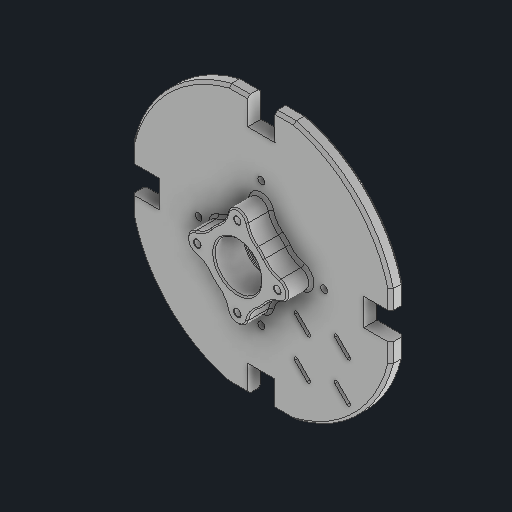
# Autodesk Inventor part: plate_lower
Saved by Autodesk Inventor 2027.1 (Build 311270010, 270A)
## iProperties
Created: 2026-10-07
Part Number: plate_lower
Material: Generisch
Document SubType Name: Modeling
Designer: luca
Density: 1 g/cm^3
Appearance: Vorgabe
Author: luca
## iProperties of the stored document plate_middle_3DPrint.ipt
Created: 2026-10-13
Part Number: plate_middle_3DPrint
Material: Generic
Document SubType Name: Modeling
Designer: lucao
Density: 1 g/cm^3
Appearance: Default
Author: lucao
Autodesk Inventor part; units mm, degrees
ref_plane "YZ Plane" through (0, 0, 0) normal (1, 0, 0) x (0, 1, 0)
ref_plane "XZ Plane" through (0, 0, 0) normal (0, 1, 0) x (-1, 0, 0)
ref_plane "XY Plane" through (0, 0, 0) normal (0, 0, 1) x (1, 0, 0)
sketch "Skizze1" plane through (0, 0, 0) normal (0, 1, 0) x (-1, 0, 0)
  circle A0 centre (0, 0) radius 100
  dimension "d0" = 200
  constraints: 1 centre point, 1 coincident
  measures "d0" diameter of A0
extrude "Extrusion1" add sketch "Skizze1" along normal blind 10
sketch "Skizze2" plane through (0, 10, 0) normal (0, 1, 0) x (1, 0, 0)
  circle A0 centre (0, 0) radius 100 projected
  circle A1 centre (-87, 0) radius 3.1
  dimension "d3" = 6.2
  dimension "d4" = 87
  dimension "d5" = 200
  constraints: 1 centre point, 1 horizontal alignment
  measures "d3" diameter of A1
  measures "d4" distance of A1.centre A0.centre
  measures "d5" diameter of A0
extrude "Extrusion2" cut sketch "Skizze2" against normal through all contours A1
chamfer "Fasen1" distance 3 angle 45 1 edges at (-90.1, 0, 0)
sketch "Skizze3" plane through (0, 10, 0) normal (0, 1, 0) x (1, 0, 0)
  circle A0 centre (-87, 0) radius 3.1 projected
  circle A1 centre (0, 0) radius 100 projected
  line L0 (-97, -24.3105) -> (-97, 24.3105)
  circle A2 centre (0, 0) radius 100 projected
  point P0 (-97, -24.3105)
  dimension "d11" = 10
  constraints: 2 end point, 1 point on circle, 1 vertical, 2 other
  measures "d11" distance from line of A0.centre L0
extrude "Extrusion3" cut sketch "Skizze3" against normal through all contours L0 A1 picked at (-97.7491, 4.0825)
pattern_circular "Runde Anordnung3" count 4 over 360 about axis through (0, -10, 0) along (0, 1, 0) of "Extrusion2", "Fasen1"
pattern_circular "Runde Anordnung4" count 4 over 360 about axis through (0, -10, 0) along (0, 1, 0) of "Extrusion3"
sketch "Skizze4" plane through (0, 0, 0) normal (0, -1, 0) x (1, 0, 0)
  circle A0 centre (0, 0) radius 15
  dimension "d26" = 30
  constraints: 1 centre point, 1 coincident
  measures "d26" diameter of A0
extrude "Extrusion4" cut sketch "Skizze4" against normal through all
sketch "Skizze5" plane through (0, 0, 0) normal (0, -1, 0) x (1, 0, 0)
  circle A0 centre (0, 0) radius 15 projected
  circle A1 centre (0, -87) radius 6.1 projected
  circle A2 centre (0, 87) radius 6.1 projected
  line L0 (-24.3105, -97) -> (24.3105, -97) projected
  arc A3 (24.3105, -97) -> (97, -24.3105) centre (0, 0) ccw projected
  line L1 (97, -24.3105) -> (97, 24.3105) projected
  arc A4 (97, 24.3105) -> (24.3105, 97) centre (0, 0) ccw projected
  line L2 (24.3105, 97) -> (-24.3105, 97) projected
  arc A5 (-24.3105, 97) -> (-97, 24.3105) centre (0, 0) ccw projected
  line L3 (-97, 24.3105) -> (-97, -24.3105) projected
  arc A6 (-97, -24.3105) -> (-24.3105, -97) centre (0, 0) ccw projected
  circle A7 centre (-87, 0) radius 6.1 projected
  circle A8 centre (87, 0) radius 6.1 projected
  line L4 (-10.25, 76.75) -> (10.25, 76.75)
  line L5 (10.25, 76.75) -> (10.25, 97.25)
  line L6 (10.25, 97.25) -> (-10.25, 97.25)
  line L7 (-10.25, 97.25) -> (-10.25, 76.75)
  line L8 (-10.25, 76.75) -> (10.25, 97.25) construction
  line L9 (10.25, 76.75) -> (-10.25, 97.25) construction
  point P0 (10.25, 97)
  point P1 (-10.25, 97)
  dimension "d29" = 20.5
  dimension "d30" = 20.5
  constraints: 12 end point, 2 midpoint, 2 parallel, 1 horizontal, 1 perpendicular
  measures "d29" distance of L6.end L5.end
  measures "d30" distance of L5.end L4.end
extrude "Extrusion5" cut sketch "Skizze5" against normal through all contours A2 | L2 L5 L4 L7
pattern_circular "Runde Anordnung5" count 4 over 360 about axis through (0, 0, 0) along (0, 1, 0) of "Extrusion5"
sketch "Sketch10" plane through (0, 0, 0) normal (0, -1, 0) x (1, 0, 0)
  circle A0 centre (0, 0) radius 25
  circle A1 centre (0, 0) radius 15 projected
  dimension "d63" = 50
  constraints: 1 centre point, 1 coincident
  measures "d63" diameter of A0
extrude "Extrusion9" add sketch "Sketch10" along normal blind 18
sketch "Sketch11" plane through (0, -18, 0) normal (0, -1, 0) x (1, 0, 0)
  circle A0 centre (0, 0) radius 17.525
  dimension "d66" = 35.05
  constraints: 1 centre point, 1 coincident
  measures "d66" diameter of A0
extrude "Extrusion10" cut sketch "Sketch11" against normal through all
sketch "Sketch12" plane through (0, 0, 0) normal (0, -1, 0) x (1, 0, 0)
  circle A0 centre (0, 0) radius 17.525 projected
  circle A1 centre (0, 0) radius 25 projected
  circle A2 centre (0, -30) radius 2.55
  circle A3 centre (0, -30) radius 7.5
  arc A4 (14.8914, -20.081) -> (7.3103, -31.6761) centre (26.8045, -36.1458) ccw
  arc A5 (-7.3103, -31.6761) -> (-14.8914, -20.081) centre (-26.8045, -36.1458) ccw
  dimension "d69" = 5.1
  dimension "d70" = 30
  dimension "d71" = 15
  dimension "d72" = 20
  dimension "d73" = 20
  constraints: 8 point on circle, 4 centre point, 4 tangent, 1 coincident, 1 vertical alignment
  measures "d69" diameter of A2
  measures "d70" distance of point (0, 0) A2.centre
  measures "d71" diameter of A3
  measures "d72" radius of A4
  measures "d73" radius of A5
extrude "Extrusion11" add sketch "Sketch12" along normal up to surface (18 mm away) contours A1 A3 A5 | A4 A3 A1 | A1 A3 picked at (2.8959, -25.9101)
pattern_circular "Circular Pattern6" count 4 over 360 about axis through (0, -18, 0) along (0, 1, 0) of "Extrusion11"
sketch "Sketch13" plane through (0, 10, 0) normal (0, 1, 0) x (1, 0, 0)
  circle A0 centre (0, 0) radius 17.525 projected
  circle A1 centre (0, 0) radius 15
  dimension "d79" = 30
  constraints: 1 centre point, 1 coincident
  measures "d79" diameter of A1
extrude "Extrusion12" add sketch "Sketch13" against normal blind 3
sketch "Sketch14" plane through (0, -18, 0) normal (0, -1, 0) x (1, 0, 0)
  circle A0 centre (30, 0) radius 2.55 projected
  circle A1 centre (0, 30) radius 2.55 projected
  circle A2 centre (-30, 0) radius 2.55 projected
  circle A3 centre (0, -30) radius 2.55 projected
  circle A4 centre (0, 0) radius 17.525 projected
  arc A5 (14.8914, -20.081) -> (20.081, -14.8914) centre (0, 0) ccw projected
  arc A6 (31.6761, -7.3103) -> (20.081, -14.8914) centre (36.1458, -26.8045) ccw projected
  arc A7 (31.6761, -7.3103) -> (31.6761, 7.3103) centre (30, 0) ccw projected
  arc A8 (20.081, 14.8914) -> (31.6761, 7.3103) centre (36.1458, 26.8045) ccw projected
  arc A9 (20.081, 14.8914) -> (14.8914, 20.081) centre (0, 0) ccw projected
  arc A10 (7.3103, 31.6761) -> (14.8914, 20.081) centre (26.8045, 36.1458) ccw projected
  arc A11 (7.3103, 31.6761) -> (-7.3103, 31.6761) centre (0, 30) ccw projected
  arc A12 (-14.8914, 20.081) -> (-7.3103, 31.6761) centre (-26.8045, 36.1458) ccw projected
  arc A13 (-14.8914, 20.081) -> (-20.081, 14.8914) centre (0, 0) ccw projected
  arc A14 (-31.6761, 7.3103) -> (-20.081, 14.8914) centre (-36.1458, 26.8045) ccw projected
  arc A15 (-31.6761, 7.3103) -> (-31.6761, -7.3103) centre (-30, 0) ccw projected
  arc A16 (-20.081, -14.8914) -> (-31.6761, -7.3103) centre (-36.1458, -26.8045) ccw projected
  arc A17 (-20.081, -14.8914) -> (-14.8914, -20.081) centre (0, 0) ccw projected
  arc A18 (-7.3103, -31.6761) -> (-14.8914, -20.081) centre (-26.8045, -36.1458) ccw projected
  arc A19 (-7.3103, -31.6761) -> (7.3103, -31.6761) centre (0, -30) ccw projected
  arc A20 (14.8914, -20.081) -> (7.3103, -31.6761) centre (26.8045, -36.1458) ccw projected
extrude "Extrusion13" cut sketch "Sketch14" against normal through all contours A0 | A1 | A2 | A3
sketch "Sketch15" plane through (0, 0, 0) normal (0, -1, 0) x (1, 0, 0)
  line L0 (0, 0) -> (70.7107, -70.7107) construction
  arc A0 (24.3105, -97) -> (97, -24.3105) centre (0, 0) ccw projected
  line L1 (0, 0) -> (0, -76.75) construction
  circle A1 centre (56.163, -56.163) radius 1.55
  circle A2 centre (26.163, -26.163) radius 1.55
  circle A3 centre (56.163, -26.163) radius 1.55
  circle A4 centre (26.163, -56.163) radius 1.55
  line L2 (26.163, -26.163) -> (56.163, -26.163) construction
  line L3 (56.163, -26.163) -> (56.163, -56.163) construction
  line L4 (56.163, -56.163) -> (26.163, -56.163) construction
  line L5 (26.163, -56.163) -> (26.163, -26.163) construction
  line L6 (26.163, -56.163) -> (35.3553, -65.3553) construction
  line L7 (56.163, -26.163) -> (65.3553, -35.3553) construction
  circle A5 centre (65.3553, -65.3553) radius 1.55
  circle A6 centre (65.3553, -35.3553) radius 1.55
  circle A7 centre (35.3553, -65.3553) radius 1.55
  circle A8 centre (35.3553, -35.3553) radius 1.55
  line L8 (55.0669, -57.259) -> (64.2593, -66.4514)
  line L9 (66.4514, -64.2593) -> (57.259, -55.0669)
  line L10 (34.2593, -66.4514) -> (25.0669, -57.259)
  line L11 (27.259, -55.0669) -> (36.4514, -64.2593)
  line L12 (34.2593, -36.4514) -> (25.0669, -27.259)
  line L13 (27.259, -25.0669) -> (36.4514, -34.2593)
  line L14 (55.0669, -27.259) -> (64.2593, -36.4514)
  line L15 (66.4514, -34.2593) -> (57.259, -25.0669)
  line L16 (-10.25, -76.75) -> (10.25, -76.75) projected
  dimension "d84" = 45
  dimension "d85" = 3.1
  dimension "d86" = 3.1
  dimension "d87" = 3.1
  dimension "d88" = 3.1
  dimension "d89" = 30
  dimension "d90" = 37
  dimension "d93" = 13
  dimension "d94" = 13
  dimension "d95" = 3.1
  dimension "d96" = 3.1
  dimension "d97" = 13
  dimension "d98" = 3.1
  dimension "d99" = 3.1
  dimension "d100" = 13
  constraints: 32 end point, 17 point on circle, 13 tangent, 8 centre point, 6 parallel, 3 coincident, 3 point on line, 2 midpoint, 1 horizontal, 1 perpendicular, 1 vertical
  measures "d84" angle of L0 L1
  measures "d85" diameter of A1
  measures "d86" diameter of A2
  measures "d87" diameter of A3
  measures "d88" diameter of A4
  measures "d89" distance of L3.end L4.end
  measures "d90" distance of L0.start L2.start
  measures "d93" distance of L4.end L6.end
  measures "d94" distance of L2.end L7.end
  measures "d95" diameter of A5
  measures "d96" diameter of A6
  measures "d97" distance of L3.end A5.centre
  measures "d98" diameter of A7
  measures "d99" diameter of A8
  measures "d100" distance of L2.start A8.centre
extrude "Extrusion14" cut sketch "Sketch15" against normal through all contours A1 | A2 | A3 | A4
extrude "Extrusion15" cut sketch "Sketch15" against normal through all contours A1 L9 A5 L8 | A5 | A2 L13 A8 L12 | A8 | A3 L15 A6 L14 | A6 | A4 L11 A7 L10 | A7
sketch "Sketch17" plane through (0, 0, 0) normal (0, -1, 0) x (1, 0, 0)
  circle A0 centre (0, -47) radius 2.6
  line L0 (-10.25, -76.75) -> (10.25, -76.75) projected
  point P0 (0, 0)
  dimension "d113" = 5.2
  dimension "d114" = 29.75
  constraints: 1 centre point, 1 vertical alignment
  measures "d113" diameter of A0
  measures "d114" distance from line of L0 A0.centre
extrude "Extrusion16" cut sketch "Sketch17" against normal through all
pattern_circular "Circular Pattern7" count 4 over 360 about axis through (0, -18, 0) along (0, 1, 0) of "Extrusion16"
fillet "Fillet3" radius 2 16 edges at (0, 0, -37.5) (17.6777, 0, -17.6777) (25.2012, 0, -10.0648) (37.5, 0, 0) (10.0648, 0, -25.2012) (17.6777, 0, 17.6777) (25.2012, 0, 10.0648) (0, 0, 37.5) (10.0648, 0, 25.2012) (-10.0648, 0, 25.2012) (-17.6777, 0, 17.6777) (-25.2012, 0, 10.0648) (-37.5, 0, 0) (-17.6777, 0, -17.6777) (-25.2012, 0, -10.0648) (-10.0648, 0, -25.2012)
chamfer "Chamfer5" distance 1 angle 45 17 edges at (25.2012, -18, -10.0648) (17.6777, -18, -17.6777) (10.0648, -18, -25.2012) (0, -18, -37.5) (-10.0648, -18, -25.2012) (-17.6777, -18, -17.6777) (-25.2012, -18, -10.0648) (-37.5, -18, 0) (-25.2012, -18, 10.0648) (-17.6777, -18, 17.6777) (-10.0648, -18, 25.2012) (0, -18, 37.5) (10.0648, -18, 25.2012) (17.6777, -18, 17.6777) (25.2012, -18, 10.0648) (37.5, -18, 0) (-17.525, -18, 0)
sketch "Sketch19" plane through (0, 0, 0) normal (1, 0, 0) x (0, 1, 0)
  line L0 (-17, -17.525) -> (7, -17.525) projected
  line L1 (7, -17.525) -> (7, 17.525) projected
  arc A0 (6.4, -18.125) -> (7, -17.525) centre (6.4, -17.525) ccw
  line L2 (6.4, -18.125) -> (5.4, -18.125)
  line L3 (5.4, -18.125) -> (4.1133, -17.525)
  line L4 (7, 0) -> (0, 0)
  dimension "d134" = 1
  dimension "d135" = 0.6
  dimension "d136" = 25
  constraints: 6 end point, 2 horizontal, 2 point on circle, 2 tangent, 1 centre point, 1 midpoint, 1 point on line
  measures "d134" distance of L2.start L2.end
  measures "d135" distance between parallel lines of L0 L2
  measures "d136" angle of L0 L3
revolve "Revolution1" cut sketch "Sketch19" angle 360 about axis through (0, 7, 0) along (0, -1, 0)
chamfer "Chamfer6" distance 0.3 angle 45 7 edges at (-28.1969, -18, -1.8031) (-31.8031, -18, 1.8031) (-2.55, -18, -30) (28.1969, -18, -1.8031) (31.8031, -18, 1.8031) (0, -18, 27.45) (0, -18, 32.55)
chamfer "Chamfer7" distance 2 angle 45 24 edges at (70.7107, 0, -70.7107) (70.7107, 10, -70.7107) (17.2802, 0, -97) (17.2802, 10, -97) (97, 0, -17.2802) (97, 10, -17.2802) (97, 0, 17.2802) (97, 10, 17.2802) (70.7107, 10, 70.7107) (70.7107, 0, 70.7107) (17.2802, 0, 97) (17.2802, 10, 97) (-17.2802, 0, 97) (-17.2802, 10, 97) (-70.7107, 0, 70.7107) (-70.7107, 10, 70.7107) (-97, 0, 17.2802) (-97, 10, 17.2802) (-97, 0, -17.2802) (-97, 10, -17.2802) (-70.7107, 0, -70.7107) (-70.7107, 10, -70.7107) (-17.2802, 0, -97) (-17.2802, 10, -97)
